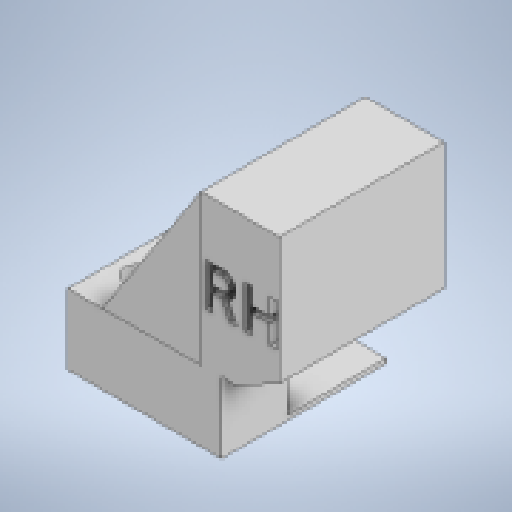
# Autodesk Inventor part: gripper
Saved by Autodesk Inventor 2024 (Build 280153000, 153)
## iProperties
Created: 2023-09-08
Part Number: gripper
Material: Generic
Document SubType Name: Modeling
Designer: 박동준
Density: 1 g/cm^3
Appearance: Default
Author: 박동준
Autodesk Inventor part; units mm, degrees
ref_plane "YZ Plane" through (0, 0, 0) normal (1, 0, 0) x (0, 1, 0)
ref_plane "XZ Plane" through (0, 0, 0) normal (0, 1, 0) x (-1, 0, 0)
sketch "Sketch1" plane through (0, 0, 0) normal (0, 0, 1) x (1, 0, 0)
  line L0 (-7.2, 32) -> (-7.2, 0)
  line L1 (-7.2, 0) -> (0, 0)
  line L2 (0, 0) -> (9.5, 5)
  line L3 (9.5, 5) -> (9.5, 32)
  line L4 (9.5, 32) -> (-7.2, 32)
  dimension "d0" = 32
  dimension "d2" = 7.2
  dimension "d55" = 9.5
  dimension "d57" = 27
  constraints: 10 end point, 2 perpendicular, 1 parallel, 1 vertical
  measures "d0" distance of L0.start L0.end
  measures "d2" distance of L0.end L1.end
  measures "d55" distance from line of L3 L1.end
  measures "d57" distance of L2.end L3.end
extrude "Extrusion1" add sketch "Sketch1" along normal mid plane 35
ref_plane "Work Plane1" through (0, 0, 15.9999) normal (0, 0, 1) x (1, 0, 0)
sketch "Sketch2" plane through (0, 0, 15.9999) normal (0, 0, 1) x (1, 0, 0)
  line L0 (-7.2, 32) -> (-7.2, 0) projected
  line L1 (-7.2, 0) -> (0, 0) projected
  line L2 (-7.2, 0) -> (-28.2, 0)
  line L3 (-7.2, 0) -> (13.8, 0) construction
  line L4 (0, 0) -> (9.5, 5) projected
  line L5 (9.5, 5) -> (9.5, 32) projected
  line L6 (9.5, 32) -> (-7.2, 32) projected
  line L7 (-28.2, 0) -> (-7.2, 32)
  line L8 (-7.2, 0) -> (-7.2, 32)
  dimension "d9" = 21
  dimension "d10" = 180
  dimension "d88" = 32
  constraints: 8 end point, 2 collinear, 2 horizontal, 1 point on line
  measures "d9" distance of L0.end L2.end
  measures "d10" angle of L2 L3
  measures "d88" distance from line of L1 L7.end
extrude "Extrusion2" add sketch "Sketch2" along normal mid plane 3 contours L0 L2 L7
mirror "Mirror1" about plane through (0, 0, 0) normal (0, 0, 1) of "Extrusion2"
sketch "Sketch3" plane through (-7.2, 0, 17.5) normal (0, -1, 0) x (1, 0, 0)
  line L0 (-42.8, 2) -> (-18.0727, 11)
  line L1 (-18.0727, 11) -> (7.2, 11)
  line L2 (7.2, 11) -> (7.2, -46)
  line L3 (-42.8, 2) -> (-42.8, -37)
  line L4 (-42.8, -37) -> (-18.0727, -46)
  line L5 (-18.0727, -46) -> (7.2, -46)
  line L6 (7.2, -35) -> (7.2, 0) projected
  line L7 (7.2, -35) -> (7.2, 0) projected
  line L8 (0, 0) -> (0, -0.0001) projected
  line L9 (7.2, -35) -> (0, -35) projected
  line L10 (0, 0) -> (7.2, 0) projected
  line L11 (-21, -0.0001) -> (0, -0.0001) projected
  line L12 (-21, -3.0001) -> (-21, -0.0001) projected
  line L13 (0, -3.0001) -> (-21, -3.0001) projected
  line L14 (0, -3.0001) -> (0, -31.9999) projected
  line L15 (0, -31.9999) -> (-21, -31.9999) projected
  line L16 (-21, -31.9999) -> (-21, -34.9999) projected
  line L17 (-21, -34.9999) -> (0, -34.9999) projected
  line L18 (0, -34.9999) -> (0, -35) projected
  point P0 (7.2, -17.5)
  point P1 (-5.4364, 11)
  point P2 (7.2, -17.5)
  point P3 (7.2, -17.5)
  point P4 (7.2, -17.5)
  point P5 (-5.4364, -46)
  point P6 (-42.8, -17.5)
  point P7 (7.2, -17.5)
  point P8 (7.2, -35)
  point P9 (7.2, 0)
  dimension "d17" = 57
  dimension "d18" = 39
  dimension "d19" = 9
  dimension "d20" = 9
  dimension "d21" = 50
  dimension "d76" = 110
  constraints: 12 end point, 7 midpoint, 3 coincident, 1 horizontal alignment, 1 perpendicular, 1 vertical alignment
  measures "d17" distance of L1.end L2.end
  measures "d18" distance of L0.start L3.end
  measures "d19" distance from line of L5 L3.end
  measures "d20" vertical distance of point (-5.436, 11) L0.start
  measures "d21" distance between parallel lines of L2 L3
  measures "d76" angle of L3 L4
extrude "Extrusion3" add sketch "Sketch3" along normal blind 16
sketch "Sketch4" plane through (-7.2, 0, 17.5) normal (0, 1, 0) x (1, 0, 0)
  line L0 (7.2, 17.5) -> (-27.8, 17.5) construction
  line L1 (-23.3, 10) -> (-3.3, 10) construction
  line L2 (-23.3, 25) -> (-23.3, 10) construction
  line L3 (7.2, 35) -> (0, 35) projected
  line L4 (7.2, 46) -> (7.2, 35) projected
  line L5 (-18.0727, 46) -> (7.2, 46) projected
  line L6 (-42.8, 37) -> (-18.0727, 46) projected
  line L7 (-42.8, -2) -> (-42.8, 37) projected
  line L8 (-18.0727, -11) -> (-42.8, -2) projected
  line L9 (7.2, -11) -> (-18.0727, -11) projected
  line L10 (7.2, 0) -> (7.2, -11) projected
  line L11 (0, 0) -> (7.2, 0) projected
  line L12 (0, 0) -> (0, 0.0001) projected
  line L13 (-21, 0.0001) -> (0, 0.0001) projected
  line L14 (-21, 3.0001) -> (-21, 0.0001) projected
  line L15 (0, 3.0001) -> (-21, 3.0001) projected
  line L16 (0, 3.0001) -> (0, 31.9999) projected
  line L17 (0, 31.9999) -> (-21, 31.9999) projected
  line L18 (-21, 31.9999) -> (-21, 34.9999) projected
  line L19 (-21, 34.9999) -> (0, 34.9999) projected
  line L20 (0, 34.9999) -> (0, 35) projected
  point P0 (-23.3, 17.5)
  point P1 (-10.3, 17.5)
  dimension "d26" = 20
  dimension "d27" = 15
  dimension "d58" = 13
  dimension "d59" = 19.5
  constraints: 6 end point, 2 horizontal, 2 midpoint, 2 perpendicular, 1 horizontal alignment
  measures "d26" distance of L1.end L1.start
  measures "d27" distance of L2.start L1.start
  measures "d58" distance from line of L2 point (-10.3, 17.5)
  measures "d59" distance from line of point (-23.3, 17.5) L7
hole "Hole1" at (-30.5, 0, 7.5) at (-10.5, 0, 7.5) at (-30.5, 0, -7.5) direction (0, -1, 0) diameter 3.1 end through all
sketch "Sketch5" plane through (0, 0, -17.5) normal (1, 0, 0) x (0, 0, -1)
  line L0 (11, 0) -> (0, 0) projected
  line L1 (-35, 0) -> (-46, 0) projected
  line L2 (-46, 0) -> (-46, -16) projected
  line L3 (11, -16) -> (-46, -16) projected
  line L4 (11, 0) -> (11, -16) projected
  line L5 (-46, 0) -> (-46, -16) projected
  line L6 (-21, -5) -> (9, -5)
  line L7 (9, -5) -> (9, -15)
  line L8 (9, -15) -> (-21, -15)
  line L9 (-21, -15) -> (-21, -5)
  line L10 (0, 0) -> (-35, 0) projected
  point P0 (-17.5, 0)
  point P1 (-17.5, 0)
  point P2 (-46, -8)
  point P3 (-46, -8)
  point P4 (11, -12.5)
  point P5 (11, -2.5)
  dimension "d46" = 30
  dimension "d47" = 10
  dimension "d48" = 2
  dimension "d49" = 5
  constraints: 8 end point, 2 midpoint, 2 parallel
  measures "d46" distance of L7.end L8.end
  measures "d47" distance of L6.end L7.end
  measures "d48" distance between parallel lines of L4 L7
  measures "d49" distance between parallel lines of L6 L0
extrude "Extrusion4" cut sketch "Sketch5" against normal blind 27 contours L6 L7 L8 L9
sketch "Sketch6" plane through (-7.2, 0, 17.5) normal (0, 1, 0) x (1, 0, 0)
  circle A0 centre (-23.3, 25) radius 1.55 projected
  circle A1 centre (-3.3, 10) radius 1.55 projected
  circle A2 centre (-23.3, 10) radius 1.55 projected
  line L0 (7.2, 35) -> (0, 35) projected
  line L1 (7.2, 46) -> (7.2, 35) projected
  line L2 (-18.0727, 46) -> (7.2, 46) projected
  line L3 (-42.8, 37) -> (-18.0727, 46) projected
  line L4 (-42.8, -2) -> (-42.8, 37) projected
  line L5 (-18.0727, -11) -> (-42.8, -2) projected
  line L6 (7.2, -11) -> (-18.0727, -11) projected
  line L7 (7.2, 0) -> (7.2, -11) projected
  line L8 (0, 0) -> (7.2, 0) projected
  line L9 (0, 0) -> (0, 0.0001) projected
  circle A3 centre (-3.3, 25) radius 2.9
  line L10 (-21, 0.0001) -> (0, 0.0001) projected
  line L11 (-21, 3.0001) -> (-21, 0.0001) projected
  line L12 (0, 3.0001) -> (-21, 3.0001) projected
  line L13 (0, 3.0001) -> (0, 31.9999) projected
  line L14 (0, 31.9999) -> (-21, 31.9999) projected
  line L15 (-21, 31.9999) -> (-21, 34.9999) projected
  line L16 (-21, 34.9999) -> (0, 34.9999) projected
  line L17 (0, 34.9999) -> (0, 35) projected
  point P0 (7.2, 17.5)
  dimension "d41" = 5.8
  dimension "d42" = 20
  dimension "d43" = 15
  constraints: 1 centre point
  measures "d41" diameter of A3
  measures "d42" distance of A3.centre A0.centre
  measures "d43" distance of A3.centre A1.centre
extrude "Extrusion5" cut sketch "Sketch6" against normal blind 3 contours A3
sketch "Sketch8" plane through (0, 0, 17.5) normal (0, 0, 1) x (1, 0, 0)
  line L0 (-7.2, 0) -> (0, 0) projected
  line L1 (0, 0) -> (9.5, 5) projected
  line L2 (9.5, 5) -> (9.5, 32) projected
  line L3 (9.5, 32) -> (-7.2, 32) projected
  line L4 (-7.2, 32) -> (-7.2, 0) projected
  line L5 (-7.2021, 20) -> (7.8, 20) construction
  line L6 (7.8, 20) -> (7.8, 7.2072) construction
  line L7 (7.8, 7.2072) -> (-7.2021, 7.2072) construction
  line L8 (-7.2021, 7.2072) -> (-7.2021, 20) construction
  line L9 (-2.756, 14.604) -> (-4.5951, 14.604)
  line L10 (-4.5951, 14.604) -> (-4.5951, 11)
  line L11 (-4.5951, 11) -> (-6.1916, 11)
  line L12 (-6.1916, 11) -> (-6.1916, 20)
  line L13 (-6.1916, 20) -> (-2.7829, 20)
  spline S0 degree 2 poles (-2.7829, 20) (-2.0823, 20) (-0.9978, 19.6228) (-0.2635, 18.976) (0.1272, 18.0666) (0.1272, 17.5277) knots 0 0 0 1 2 3 4 4 4
  line L14 (0.1272, 17.5277) -> (0.1272, 17.0629)
  spline S1 degree 2 poles (0.1272, 17.0629) (0.1272, 16.3555) (-0.5734, 15.2171) (-1.274, 14.9072) knots 0 0 0 1 2 2 2
  spline S2 degree 2 poles (-1.274, 14.9072) (-0.8226, 13.9169) (0.0397, 11.9835) (0.4843, 11) knots 0 0 0 1 2 2 2
  line L15 (0.4843, 11) -> (-1.247, 11)
  line L16 (-1.247, 11) -> (-2.756, 14.604)
  line L17 (-4.5951, 18.6662) -> (-4.5951, 15.9446)
  line L18 (-4.5951, 15.9446) -> (-3.1198, 15.9446)
  spline S3 degree 2 poles (-3.1198, 15.9446) (-2.1969, 15.9446) (-1.4626, 16.5913) (-1.4626, 17.1033) knots 0 0 0 1 2 2 2
  line L19 (-1.4626, 17.1033) -> (-1.4626, 17.4805)
  spline S4 degree 2 poles (-1.4626, 17.4805) (-1.4626, 17.9993) (-2.1564, 18.6662) (-2.985, 18.6662) knots 0 0 0 1 2 2 2
  line L20 (-2.985, 18.6662) -> (-4.5951, 18.6662)
  line L21 (7.3757, 15.0284) -> (3.6437, 15.0284)
  line L22 (3.6437, 15.0284) -> (3.6437, 11)
  line L23 (3.6437, 11) -> (2.0472, 11)
  line L24 (2.0472, 11) -> (2.0472, 20)
  line L25 (2.0472, 20) -> (3.6437, 20)
  line L26 (3.6437, 20) -> (3.6437, 16.3555)
  line L27 (3.6437, 16.3555) -> (7.3757, 16.3555)
  line L28 (7.3757, 16.3555) -> (7.3757, 20)
  line L29 (7.3757, 20) -> (8.979, 20)
  line L30 (8.979, 20) -> (8.979, 11)
  line L31 (8.979, 11) -> (7.3757, 11)
  line L32 (7.3757, 11) -> (7.3757, 15.0284)
  point P0 (-7, 15)
  dimension "d68" = 12
  dimension "d69" = 15
  constraints: 2 other
  measures "d68" distance between parallel lines of L5 L3
  measures "d69" distance between parallel lines of L6 L4
extrude "Extrusion7" cut sketch "Sketch8" against normal blind 5 contours L9 L10 L11 L12 L13 S0 L14 S1 S2 L15 L16 | L21 L22 L23 L24 L25 L26 L27 L28 L29 L30 L31 L32
sketch "Sketch9" plane through (0, 0, -17.5) normal (0, 0, -1) x (-1, 0, 0)
  line L0 (-2.0472, 11) -> (-2.0472, 20) projected
  line L1 (0, 0) -> (7.2, 0) projected
  line L2 (7.2, 0) -> (7.2, 32) projected
  line L3 (7.2, 32) -> (-9.5, 32) projected
  line L4 (-9.5, 32) -> (-9.5, 5) projected
  line L5 (-9.5, 5) -> (0, 0) projected
  line L6 (-8.356, 20) -> (-4.8532, 20) construction
  line L7 (-4.8532, 20) -> (-4.8532, 17.8281) construction
  line L8 (-4.8532, 17.8281) -> (-8.356, 17.8281) construction
  line L9 (-8.356, 17.8281) -> (-8.356, 20) construction
  line L10 (5.5, 50.4054) -> (5.5, 41.2692)
  line L11 (5.0759, 13.3023) -> (-0.0051, 13.3023)
  line L12 (-0.0051, 13.3023) -> (-0.0051, 8.2212)
  line L13 (-0.0051, 8.2212) -> (-1.6826, 8.2212)
  line L14 (-1.6826, 8.2212) -> (-1.6826, 13.3023)
  line L15 (-1.6826, 13.3023) -> (-6.7636, 13.3023)
  line L16 (-6.7636, 13.3023) -> (-6.7636, 14.919)
  line L17 (-6.7636, 14.919) -> (-1.6826, 14.919)
  line L18 (-1.6826, 14.919) -> (-1.6826, 20)
  line L19 (-1.6826, 20) -> (-0.0051, 20)
  line L20 (-0.0051, 20) -> (-0.0051, 14.919)
  line L21 (-0.0051, 14.919) -> (5.0759, 14.919)
  line L22 (5.0759, 14.919) -> (5.0759, 13.3023)
  dimension "d72" = 12
  dimension "d73" = 15
  constraints: 2 end point, 1 vertical, 2 other
  measures "d72" distance between parallel lines of L3 L6
  measures "d73" distance between parallel lines of L10 L4
extrude "Extrusion8" cut sketch "Sketch9" against normal blind 5 contours L15 L16 L17 L0 | L0 L17 L18 L19 L20 L21 L22 L11 L12 L13 L14 L15
sketch "Sketch10" plane through (-7.2, 0, 17.5) normal (0, 1, 0) x (1, 0, 0)
  line L0 (-30.65, 19.5) -> (4.05, 19.5) projected
  circle A0 centre (-23.3, 25) radius 1.55 projected
  circle A1 centre (-23.3, 10) radius 1.55 projected
  circle A2 centre (-3.3, 10) radius 1.55 projected
  circle A3 centre (-23.3, 25) radius 2.9
  circle A4 centre (-23.3, 10) radius 2.9
  circle A5 centre (-3.3, 10) radius 2.9
  point P0 (7.2, 17.5)
  dimension "d77" = 5.8
  dimension "d78" = 5.8
  dimension "d79" = 5.8
  constraints: 3 centre point, 3 coincident
  measures "d77" diameter of A3
  measures "d78" diameter of A4
  measures "d79" diameter of A5
extrude "Extrusion9" cut sketch "Sketch10" against normal blind 10 contours A0 | A1 | A3 | A4 | A5
sketch "Sketch12" plane through (-7.2, 0, 17.5) normal (0, 1, 0) x (1, 0, 0)
  circle A0 centre (-3.3, 25) radius 2.9 projected
  circle A1 centre (-3.3, 25) radius 1.55
  point P0 (7.2, 17.5)
  dimension "d85" = 3.1
  constraints: 2 coincident, 1 centre point
  measures "d85" diameter of A1
extrude "Extrusion11" cut sketch "Sketch12" against normal blind 4 contours A1
sketch "Sketch13" plane through (-7.2, 0, 17.5) normal (0, 1, 0) x (1, 0, 0)
  circle A0 centre (-3.3, 10) radius 2.9 projected
  circle A1 centre (-23.3, 25) radius 2.9 projected
  circle A2 centre (-23.3, 10) radius 2.9 projected
  circle A3 centre (-3.3, 25) radius 2.9 projected
  line L0 (7.2, 35) -> (0, 35) projected
  line L1 (7.2, 46) -> (7.2, 35) projected
  line L2 (-18.0727, 46) -> (7.2, 46) projected
  line L3 (-42.8, 37) -> (-18.0727, 46) projected
  line L4 (-42.8, -2) -> (-42.8, 37) projected
  line L5 (-18.0727, -11) -> (-42.8, -2) projected
  line L6 (7.2, -11) -> (-18.0727, -11) projected
  line L7 (7.2, 0) -> (7.2, -11) projected
  line L8 (0, 0) -> (7.2, 0) projected
  line L9 (0, 0) -> (0, 0.0001) projected
  line L10 (-21, 0.0001) -> (0, 0.0001) projected
  line L11 (-21, 3.0001) -> (-21, 0.0001) projected
  line L12 (0, 3.0001) -> (-21, 3.0001) projected
  line L13 (0, 3.0001) -> (0, 31.9999) projected
  line L14 (0, 31.9999) -> (-21, 31.9999) projected
  line L15 (-21, 31.9999) -> (-21, 34.9999) projected
  line L16 (-21, 34.9999) -> (0, 34.9999) projected
  line L17 (0, 34.9999) -> (0, 35) projected
  line L18 (7.2, -11) -> (-42.8, -11)
  line L19 (-42.8, -11) -> (-42.8, 0)
  line L20 (-42.8, 0) -> (7.2, 0)
  line L21 (7.2, 0) -> (7.2, -11)
  line L22 (7.2, 46) -> (-42.8, 46)
  line L23 (-42.8, 46) -> (-42.8, 35)
  line L24 (-42.8, 35) -> (7.2, 35)
  line L25 (7.2, 35) -> (7.2, 46)
  point P0 (7.2, 17.5)
  point P1 (7.2, 40.5)
  dimension "d89" = 11
  dimension "d92" = 11
  dimension "d93" = 50
  constraints: 16 end point, 4 parallel, 2 horizontal, 2 perpendicular, 1 midpoint, 1 point on line
  measures "d89" distance between parallel lines of L18 L20
  measures "d92" distance between parallel lines of L2 L24
  measures "d93" distance from line of point (7.2, 40.5) L23
extrude "Extrusion12" cut sketch "Sketch13" against normal blind 30 contours L0 L16 L24 L4 L3 L2 L1 | L20 L10 L8 L7 L6 L5 L4
sketch "Sketch14" plane through (-7.2, 0, 17.5) normal (0, 1, 0) x (1, 0, 0)
  line L0 (-42.8, 0) -> (0, 0) projected
  line L1 (0, 0) -> (0, 0.0001) projected
  line L2 (-21, 0.0001) -> (0, 0.0001) projected
  line L3 (-21, 3.0001) -> (-21, 0.0001) projected
  line L4 (0, 3.0001) -> (-21, 3.0001) projected
  line L5 (0, 3.0001) -> (0, 31.9999) projected
  line L6 (0, 31.9999) -> (-21, 31.9999) projected
  line L7 (-21, 31.9999) -> (-21, 34.9999) projected
  line L8 (-21, 34.9999) -> (0, 34.9999) projected
  line L9 (0, 34.9999) -> (0, 35) projected
  line L10 (0, 35) -> (-42.8, 35) projected
  line L11 (-42.8, 0) -> (-42.8, 35) projected
  circle A0 centre (-3.3, 10) radius 2.9 projected
  circle A1 centre (-23.3, 25) radius 2.9 projected
  circle A2 centre (-23.3, 10) radius 2.9 projected
  circle A3 centre (-3.3, 25) radius 2.9 projected
  line L12 (-42.8, 0) -> (-28.3, 0)
  line L13 (-28.3, 0) -> (-28.3, 35)
  line L14 (-28.3, 35) -> (-42.8, 35)
  line L15 (-42.8, 35) -> (-42.8, 0)
  point P0 (7.2, 17.5)
  point P1 (-28.3, 0)
  dimension "d94" = 5
  constraints: 8 end point, 2 parallel, 1 horizontal, 1 perpendicular, 1 point on line
  measures "d94" distance from line of L13 A1.centre
extrude "Extrusion13" cut sketch "Sketch14" against normal through all contours L11 L10 L13 L0
sketch "Sketch15" plane through (0, 0, 17.5) normal (0, 0, 1) x (1, 0, 0)
  line L0 (-1.247, 11) -> (-2.756, 14.604) projected
  line L1 (-2.756, 14.604) -> (-4.5951, 14.604) projected
  line L2 (-4.5951, 14.604) -> (-4.5951, 11) projected
  line L3 (-4.5951, 11) -> (-6.1916, 11) projected
  line L4 (-6.1916, 11) -> (-6.1916, 20) projected
  line L5 (-6.1916, 20) -> (-2.7829, 20) projected
  line L6 (0.1272, 17.5277) -> (0.1272, 17.0629) projected
  line L7 (0.4843, 11) -> (-1.247, 11) projected
  line L8 (7.3757, 11) -> (7.3757, 15.0284) projected
  line L9 (7.3757, 15.0284) -> (3.6437, 15.0284) projected
  line L10 (3.6437, 15.0284) -> (3.6437, 11) projected
  line L11 (3.6437, 11) -> (2.0472, 11) projected
  line L12 (2.0472, 11) -> (2.0472, 20) projected
  line L13 (2.0472, 20) -> (3.6437, 20) projected
  line L14 (3.6437, 20) -> (3.6437, 16.3555) projected
  line L15 (3.6437, 16.3555) -> (7.3757, 16.3555) projected
  line L16 (7.3757, 16.3555) -> (7.3757, 20) projected
  line L17 (7.3757, 20) -> (8.979, 20) projected
  line L18 (8.979, 20) -> (8.979, 11) projected
  line L19 (8.979, 11) -> (7.3757, 11) projected
  line L20 (-35.5, 0) -> (-35.5, -16) projected
  line L21 (0, -16) -> (-35.5, -16) projected
  line L22 (0, 0) -> (0, -16) projected
  line L23 (0, 0) -> (9.5, 5) projected
  line L24 (9.5, 5) -> (9.5, 32) projected
  line L25 (9.5, 32) -> (-7.2, 32) projected
  line L26 (-7.2, 32) -> (-7.2, 0) projected
  line L27 (-35.5, 0) -> (-7.2, 0) projected
  line L28 (0, 0) -> (-2.8, 0)
  line L29 (-2.8, 0) -> (-2.8, -16)
  line L30 (-2.8, -16) -> (0, -16)
  line L31 (0, -16) -> (0, 0)
  dimension "d97" = 2.8
  constraints: 8 end point, 2 parallel, 1 horizontal, 1 perpendicular, 1 point on line, 3 other
  measures "d97" distance of L29.end L30.end
extrude "Extrusion14" cut sketch "Sketch15" against normal up to surface (35 mm away) contours L29 L28 L22 L21
body "Solid1"
